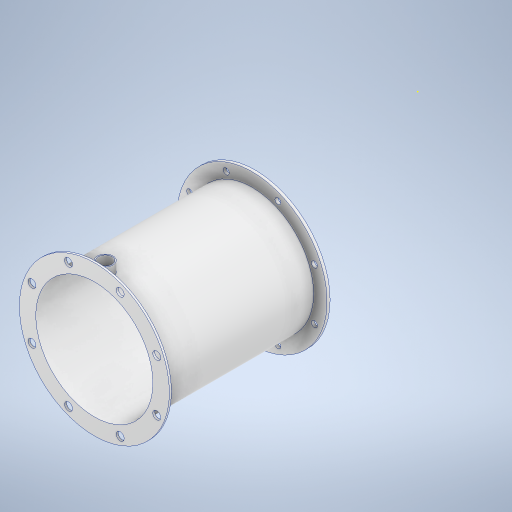
# Autodesk Inventor part: aluminium outer wall - front
Saved by Autodesk Inventor 2023 (Build 270158000, 158)
## iProperties
Created: 2022-09-19
Part Number: aluminium outer wall - front
Material: Aluminum 6061
Document SubType Name: Modeling
Designer: station
Density: 2.7 g/cm^3
Appearance: Aluminum - Flat
Author: station
Autodesk Inventor part; units mm, degrees
ref_plane "YZ Plane" through (0, 0, 0) normal (1, 0, 0) x (0, 1, 0)
ref_plane "XY Plane" through (0, 0, 0) normal (0, 0, 1) x (1, 0, 0)
sketch "Sketch1" plane through (0, 0, 0) normal (0, 0, 1) x (1, 0, 0)
  circle A0 centre (0, 0) radius 58.5
  circle A1 centre (0, 0) radius 61.5
  dimension "d0" = 117
  dimension "d1" = 123
  constraints: 2 centre point, 2 coincident
  measures "d0" diameter of A0
  measures "d1" diameter of A1
extrude "Extrusion1" add sketch "Sketch1" along normal blind 323.123
ref_plane "Work Plane1" through (0, 61.5, 0) normal (0, 1, 0) x (-1, 0, 0)
sketch "Sketch2" plane through (0, 61.5, 0) normal (0, 1, 0) x (-1, 0, 0)
  line L0 (61.5, 0) -> (-61.5, 0) projected
  line L1 (0, 0) -> (0, 4)
  line L2 (0, 4) -> (0, 8.666)
  circle A0 centre (0, 15.524) radius 6.858
  circle A1 centre (0, 15.524) radius 7.858
  dimension "d6" = 4
  dimension "d7" = 4.666
  dimension "d8" = 13.716
  dimension "d9" = 6.858
  dimension "d33" = 15.716
  constraints: 4 end point, 2 centre point, 1 coincident, 1 point on line, 1 vertical
  measures "d6" distance of L1.start L1.end
  measures "d7" distance of L1.end L2.end
  measures "d8" diameter of A0
  measures "d9" distance of A0.centre L2.end
  measures "d33" diameter of A1
extrude "Extrusion2" cut sketch "Sketch2" against normal blind 23 contours A0
sketch "Sketch3" plane through (0, 61.5, 0) normal (0, 1, 0) x (-1, 0, 0)
  line L0 (0, 0) -> (0, 323.123) construction
  line L1 (-58.5, 323.123) -> (58.5, 323.123) projected
  line L2 (0, 323.123) -> (0, 315.123) construction
  circle A0 centre (0, 312.265) radius 6.858
  circle A1 centre (0, 312.265) radius 7.858
  point P0 (0, 319.123)
  dimension "d12" = 8
  dimension "d13" = 13.716
  dimension "d14" = 6.858
  dimension "d36" = 15.716
  constraints: 4 end point, 2 centre point, 2 midpoint, 2 point on line, 1 coincident
  measures "d12" distance of L0.end L2.end
  measures "d13" diameter of A0
  measures "d14" distance of A0.centre point (0, 319.123)
  measures "d36" diameter of A1
extrude "Extrusion3" cut sketch "Sketch3" against normal blind 3 contours A0
thread "Thread1" size "M14x1.25" class "6H" standard "ANSI Metric M Profile" full length
thread "Thread2" size "M14x1.25" class "6H" standard "ANSI Metric M Profile" full length
sketch "Sketch4" plane through (0, 61.5, 0) normal (0, 1, 0) x (-1, 0, 0)
  point P0 (0, 0)
sketch "Sketch5" plane through (0, 61.5, 0) normal (0, 1, 0) x (-1, 0, 0)
  line L0 (0, 0) -> (0, 76) construction
  circle A0 centre (0, 76) radius 4
  dimension "d21" = 76
  dimension "d22" = 8
  constraints: 2 end point, 1 centre point, 1 coincident, 1 vertical
  measures "d21" distance of L0.start L0.end
  measures "d22" diameter of A0
extrude "Extrusion4" cut sketch "Sketch5" against normal through all
thread "Thread3" size "M8x1.25" class "6H" standard "ANSI Metric M Profile" full length
thread "Thread4" size "M8x1.25" class "6H" standard "ANSI Metric M Profile" full length
sketch "Sketch6" plane through (0, 0, 323.123) normal (0, 0, 1) x (1, 0, 0)
  circle A0 centre (0, 0) radius 75
  circle A1 centre (0, 0) radius 61.5
  dimension "d29" = 150
  dimension "d30" = 123
  constraints: 2 centre point, 2 coincident
  measures "d29" diameter of A0
  measures "d30" diameter of A1
extrude "Extrusion5" add sketch "Sketch6" against normal blind 2
extrude "Extrusion6" add sketch "Sketch2" along normal blind 10
extrude "Extrusion7" add sketch "Sketch3" along normal blind 10
ref_plane "Work Plane2" through (0, 0, 162.5) normal (0, 0, -1) x (-1, 0, 0)
sketch "Sketch7" plane through (0, 0, 162.5) normal (0, 0, -1) x (-1, 0, 0)
  circle A0 centre (0, 0) radius 75
  circle A1 centre (0, 0) radius 58.5 projected
  circle A2 centre (0, 0) radius 59.5
  dimension "d40" = 150
  constraints: 2 centre point, 2 coincident
  measures "d40" diameter of A0
extrude "Extrusion10" add sketch "Sketch7" along normal blind 3 contours A0 | A2
extrude "Extrusion11" add sketch "Sketch7" against normal blind 3 contours A0 | A2
split "Split3" plane through (0, 0, 162.5) removes the side toward (0, 0, -1)
sketch "Sketch8" plane through (0, 0, 323.123) normal (0, 0, 1) x (1, 0, 0)
  line L0 (0, 0) -> (0, 98.0779) construction
  line L1 (0, 0) -> (25.8311, 62.3619) construction
  circle A0 centre (25.8311, 62.3619) radius 4
  line L2 (0, 0) -> (62.3619, 25.8311) construction
  circle A1 centre (62.3619, 25.8311) radius 4
  line L3 (0, 0) -> (62.3619, -25.8311) construction
  circle A2 centre (62.3619, -25.8311) radius 4
  line L4 (0, 0) -> (25.8311, -62.3619) construction
  circle A3 centre (25.8311, -62.3619) radius 4
  line L5 (0, 0) -> (-25.8311, -62.3619) construction
  circle A4 centre (-25.8311, -62.3619) radius 4
  line L6 (0, 0) -> (-62.3619, -25.8311) construction
  circle A5 centre (-62.3619, -25.8311) radius 4
  line L7 (0, 0) -> (-62.3619, 25.8311) construction
  circle A6 centre (-62.3619, 25.8311) radius 4
  line L8 (0, 0) -> (-25.8311, 62.3619) construction
  circle A7 centre (-25.8311, 62.3619) radius 4
  dimension "d49" = 22.5
  dimension "d50" = 67.5
  dimension "d51" = 8
  dimension "d54" = 360
  constraints: 18 end point, 10 coincident, 8 centre point, 1 vertical, 39 other
  measures "d49" angle of L1 L0
  measures "d50" distance of L0.start L1.end
  measures "d51" diameter of A0
hole "Hole1" at (25.8311, 62.3619, 323.123) at (-25.8311, 62.3619, 323.123) at (-62.3619, 25.8311, 323.123) at (-62.3619, -25.8311, 323.123) at (62.3619, 25.8311, 323.123) at (62.3619, -25.8311, 323.123) at (25.8311, -62.3619, 323.123) at (-25.8311, -62.3619, 323.123) direction (0, 0, -1) diameter 8 depth 2 tip angle 118
sketch "Sketch9" plane through (0, 0, 162.5) normal (0, 0, -1) x (-1, 0, 0)
  line L0 (0, 0) -> (0, 103.9992)
  line L1 (0, 0) -> (25.8311, 62.3619)
  circle A0 centre (25.8311, 62.3619) radius 4 projected
  circle A1 centre (25.8311, 62.3619) radius 3
  circle A2 centre (-25.8311, 62.3619) radius 3
  circle A3 centre (-62.3619, 25.8311) radius 3
  circle A4 centre (-62.3619, -25.8311) radius 3
  circle A5 centre (-25.8311, -62.3619) radius 3
  circle A6 centre (25.8311, -62.3619) radius 3
  circle A7 centre (62.3619, -25.8311) radius 3
  circle A8 centre (62.3619, 25.8311) radius 3
  dimension "d63" = 22.5
  dimension "d64" = 67.5
  dimension "d65" = 6
  dimension "d68" = 360
  constraints: 8 centre point, 4 end point, 3 coincident, 1 vertical, 23 other
  measures "d63" angle of L1 L0
  measures "d64" distance of L0.start L1.end
  measures "d65" diameter of A1
hole "Hole2" at (-25.8311, 62.3619, 162.5) at (25.8311, 62.3619, 162.5) at (62.3619, 25.8311, 162.5) at (62.3619, -25.8311, 162.5) at (25.8311, -62.3619, 162.5) at (-25.8311, -62.3619, 162.5) at (-62.3619, -25.8311, 162.5) at (-62.3619, 25.8311, 162.5) direction (0, 0, 1) diameter 6 depth 3 tip angle 118
body "Solid1"
